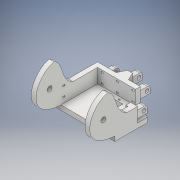
# Autodesk Inventor part: palm
Saved by Autodesk Inventor 2018 (Build 220112000, 112)
## iProperties
Created: 2018-02-09
Part Number: palm
Material: Plastique ABS
Document SubType Name: Modeling
Designer: Thomas
Density: 1.06 g/cm^3
Appearance: Lisse - Blanc
Author: Thomas
Autodesk Inventor part; units mm, degrees
ref_plane "YZ Plane" through (0, 0, 0) normal (1, 0, 0) x (0, 1, 0)
ref_plane "XZ Plane" through (0, 0, 0) normal (0, 1, 0) x (-1, 0, 0)
ref_plane "XY Plane" through (0, 0, 0) normal (0, 0, 1) x (1, 0, 0)
sketch "Esquisse1" plane through (0, 0, 0) normal (0, 0, 1) x (1, 0, 0)
  line L0 (0, 0) -> (44.9, 0)
  line L1 (44.9, 0) -> (44.9, 5)
  line L2 (0, 5) -> (0, 0)
  line L3 (23.4, 13) -> (28.6, 13)
  line L4 (28.6, 13) -> (32.5, 5)
  line L5 (23.4, 13) -> (19.5, 5)
  line L6 (0, 5) -> (19.5, 5)
  line L7 (32.5, 5) -> (44.9, 5)
  line L8 (28.6, 13) -> (28.6, 5) construction
  line L9 (28.6, 5) -> (32.5, 5) construction
  line L10 (23.4, 13) -> (23.4, 5) construction
  line L11 (23.4, 5) -> (19.5, 5) construction
  dimension "d0" = 5
  dimension "d1" = 44.9
  dimension "d2" = 13
  dimension "d3" = 13
  dimension "d5" = 5.2
  dimension "d146" = 3.9
  dimension "d147" = 3.9
  dimension "d148" = 12.4
  constraints: 24 end point, 4 horizontal, 2 perpendicular, 1 collinear, 1 parallel, 1 vertical
  measures "d0" distance of L0.end L1.end
  measures "d1" distance of L1.end L2.start
  measures "d2" distance of L4.end L5.end
  measures "d3" distance between parallel lines of L0 L3
  measures "d5" distance of L3.start L3.end
  measures "d146" distance of L8.end L4.end
  measures "d147" distance of L10.end L5.end
  measures "d148" distance of L4.end L1.end
extrude "Extrusion1" add sketch "Esquisse1" along normal blind 15
sketch "Esquisse2" plane through (44.9, 0, 0) normal (1, 0, 0) x (0, 0, -1)
  line L0 (0, 0) -> (-15, 0) projected
  line L1 (0, 0) -> (-15, 0)
  line L2 (-15, 0) -> (-15, -19.5)
  line L3 (-15, -19.5) -> (0, -19.5)
  line L4 (0, -19.5) -> (0, 0)
  point P0 (-15, 5)
  dimension "d11" = 19.5
  dimension "d18" = 15
  constraints: 8 end point, 2 parallel, 1 horizontal, 1 perpendicular
  measures "d11" distance of L3.end L0.start
  measures "d18" distance of L2.end L3.end
extrude "Extrusion2" add sketch "Esquisse2" against normal blind 5
sketch "Esquisse3" plane through (44.9, -19.5, 0) normal (0, -1, 0) x (1, 0, 0)
  line L0 (0, 0) -> (0, 15) projected
  line L1 (0, 15) -> (16.5, 15)
  line L2 (16.5, 15) -> (16.5, 0)
  line L3 (16.5, 0) -> (0, 0)
  line L4 (0, 0) -> (0, 15)
  point P0 (-44.9, 0)
  dimension "d14" = 16.5
  dimension "d19" = 15
  constraints: 8 end point, 2 parallel, 1 horizontal, 1 perpendicular
  measures "d14" distance of L2.end L3.end
  measures "d19" distance of L1.end L2.end
extrude "Extrusion3" add sketch "Esquisse3" against normal blind 5
sketch "Esquisse5" plane through (61.4, -19.5, 15) normal (1, 0, 0) x (0, 0, -1)
  line L0 (0, 0) -> (0, 19.5) projected
  spline S0 degree 3 poles (15, -18.85) (12.4289, -60.7765) (-25.3218, -44.0983) (-27.81, -26.0736) knots 0 0 0 0 1 1 1 1
  line L1 (0, 0) -> (-12.0102, 0) construction
  spline S1 degree 3 poles (0, -6.5) (-6.4739, -20.1212) (-23.0066, -15.548) (-27.81, -26.0736) knots 0 0 0 0 1 1 1 1
  line L2 (15, 0) -> (0, 0)
  line L3 (15, 19.5) -> (15, 0) projected
  line L4 (15, -18.85) -> (15, 0)
  line L5 (15, 0) -> (0, 0) projected
  line L6 (15, 0) -> (0, 0)
  line L7 (0, 0) -> (0, -6.5)
  line L8 (0, -26) -> (-10, -26) construction
  circle A0 centre (-5, -26) radius 5 construction
  point P0 (-0.0048, -44.59)
  point P1 (-18.0068, -40.3478)
  point P2 (-9.9873, -15.735)
  point P3 (-20.8554, -19.7545)
  dimension "d21" = 6.5
  dimension "d24" = 10
  dimension "d26" = 26
  dimension "d27" = 26
  dimension "d28" = 44.59
  dimension "d31" = 17.81
  dimension "d32" = 10
  constraints: 12 end point, 2 horizontal, 1 centre point, 1 collinear, 1 midpoint, 1 perpendicular, 1 vertical, 8 other
  measures "d21" distance of L0.start L7.end
  measures "d24" distance of L8.end L8.start
  measures "d26" distance of L0.start L8.start
  measures "d27" distance from line of L1 L8.end
  measures "d28" distance of point (-0.005, -44.59) L0.start
  measures "d31" horizontal distance of point (-27.81, -26.074) L8.end
  measures "d32" diameter of A0
extrude "Extrusion4" add sketch "Esquisse5" against normal blind 5
sketch "Esquisse6" plane through (61.4, -14.5, 15) normal (1, 0, 0) x (0, 0, -1)
  circle A0 centre (-5.6857, -35.9029) radius 2.6
  point P0 (15, 14.5)
  point P1 (0, 0)
  dimension "d213" = 5.2
  constraints: 1 centre point, 1 coincident
  measures "d213" diameter of A0
extrude "Extrusion5" cut sketch "Esquisse6" against normal blind 5
sketch "Esquisse7" plane through (0, 0, 0) normal (-1, 0, 0) x (0, 0, 1)
  line L0 (15, -19.4715) -> (15, 0)
  spline S0 degree 3 poles (0, -38.3215) (2.8582, -79.9664) (39.8923, -64.0148) (42.81, -45.5451) knots 0 0 0 0 1 1 1 1
  line L1 (15, -19.4715) -> (27.0102, -19.4715) construction
  spline S1 degree 3 poles (15, -25.9715) (21.48, -39.5796) (38.0003, -35.0338) (42.81, -45.5451) knots 0 0 0 0 1 1 1 1
  line L2 (0, 0) -> (0, -19.4715)
  line L3 (0, -38.3215) -> (0, -19.4715)
  line L4 (15, -19.4715) -> (15, -25.9715)
  line L5 (15, -45.4715) -> (25, -45.4715) construction
  circle A0 centre (20, -45.4715) radius 5 construction
  line L6 (15, 0) -> (0, 0)
  line L7 (0, 0) -> (15, 0) projected
  line L8 (15, -19.5) -> (15, 0) projected
  line L9 (0, 0) -> (0, -19.5) projected
  line L10 (0, -19.5) -> (15, -19.5) construction
  line L11 (15, -19.5) -> (15, -70.8185) construction
  point P0 (15, -26)
  point P1 (15, -64.0615)
  point P2 (32.7077, -60.0762)
  point P3 (24.9887, -35.2044)
  point P4 (35.8544, -39.2301)
  point P5 (42.81, -45.5736)
  dimension "d62" = 0
  dimension "d63" = 0
  dimension "d64" = 0
  dimension "d66" = 17.81
  dimension "d67" = 44.59
  dimension "d68" = 0
  dimension "d69" = 10
  dimension "d70" = 5
  dimension "d71" = 0
  constraints: 16 end point, 1 centre point, 1 horizontal, 1 vertical, 8 other
  measures "d62" distance between parallel lines of L7 L6
  measures "d63" distance between parallel lines of L0 L8
  measures "d64" distance between parallel lines of L2 L9
  measures "d66" horizontal distance of point (42.81, -45.545) L5.end
  measures "d67" distance of point (15, -64.062) L1.start
  measures "d68" distance from line of L11 L5.start
  measures "d69" diameter of A0
  measures "d70" distance of L5.start A0.centre
  measures "d71" distance from line of L11 point (15, -64.062)
extrude "Extrusion6" add sketch "Esquisse7" against normal blind 5
sketch "Esquisse9" plane through (0, 5, 0) normal (-1, 0, 0) x (0, 0, 1)
  line L0 (0, 0) -> (15, 0) construction
  line L1 (15, 0) -> (15, -38) construction
  line L2 (15, -38) -> (7.2, -38)
  line L3 (7.2, -38) -> (7.2, -43.2)
  line L4 (7.2, -43.2) -> (15, -43.2)
  line L5 (15, -43.2) -> (15, -38)
  point P0 (0, -5)
  dimension "d76" = 38
  dimension "d78" = 7.8
  dimension "d79" = 5.2
  constraints: 10 end point, 2 vertical, 1 horizontal, 1 parallel, 1 perpendicular
  measures "d76" distance of L0.end L1.end
  measures "d78" distance of L1.end L2.end
  measures "d79" distance of L2.end L3.end
extrude "Extrusion8" add sketch "Esquisse9" along normal blind 10.4
sketch "Esquisse10" plane through (0, -33, 15) normal (0, 1, 0) x (1, 0, 0)
  circle A0 centre (-6.9337, 3.9) radius 2
  arc A1 (-10.4, 3) -> (-7.4, 0) centre (-7.4, 3) ccw construction
  line L0 (-10.4, 3) -> (-10.4, 10.1049) construction
  line L1 (-10.4, 10.1049) -> (-10.4, -0.5302) construction
  line L2 (0, 0) -> (-10.4, 0) construction
  line L3 (0, 7.8) -> (0, 0) construction
  line L4 (0, 7.8) -> (-10.4, 7.8) construction
  line L5 (-3.4673, 0) -> (-3.4673, 7.8) construction
  line L6 (-10.4, 0) -> (-3.4673, 7.8) construction
  line L7 (-3.4673, 0) -> (-10.4, 7.8) construction
  point P0 (0, 15)
  dimension "d84" = 4
  dimension "d111" = 3.4674
  constraints: 14 end point, 5 point on line, 3 perpendicular, 1 centre point, 1 midpoint, 1 point on circle, 1 tangent, 1 vertical
  measures "d84" diameter of A0
  measures "d111" distance between parallel lines of L3 L5
extrude "Extrusion9" cut sketch "Esquisse10" against normal blind 5.2
sketch "Esquisse11" plane through (0, 5, 0) normal (-1, 0, 0) x (0, 0, 1)
  line L0 (11.1472, -39.2716) -> (11.1472, -43.1725)
  line L1 (7.2, -38) -> (15, -38) projected
  line L2 (14.1279, -41.7) -> (14.1279, -39.5)
  line L3 (15, -38) -> (15, -43.2) projected
  line L4 (17, -41.7) -> (15.5, -41.7)
  line L5 (15.5, -41.7) -> (15.5, -39.5)
  line L6 (15.5, -39.5) -> (17, -39.5)
  line L7 (17, -39.5) -> (17, -41.7)
  line L8 (6.7, -41.7) -> (5.2, -41.7)
  line L9 (5.2, -41.7) -> (5.2, -39.5)
  line L10 (5.2, -39.5) -> (6.7, -39.5)
  line L11 (6.7, -39.5) -> (6.7, -41.7)
  line L12 (7.2, -43.2) -> (7.2, -38) projected
  point P0 (0, -5)
  dimension "d93" = 0.5
  dimension "d94" = 1.5
  dimension "d95" = 1.5
  dimension "d96" = 2.2
  dimension "d97" = 2.2
  dimension "d98" = 1.5
  dimension "d99" = 0.5
  dimension "d100" = 1.5
  constraints: 20 end point, 4 parallel, 2 horizontal, 2 perpendicular
  measures "d93" distance between parallel lines of L3 L5
  measures "d94" distance of L5.end L6.end
  measures "d95" distance between parallel lines of L6 L1
  measures "d96" distance of L6.end L4.start
  measures "d97" distance of L8.end L9.end
  measures "d98" distance of L9.end L10.end
  measures "d99" distance between parallel lines of L12 L11
  measures "d100" distance between parallel lines of L1 L10
extrude "Extrusion11" cut sketch "Esquisse11" against normal blind 5
sketch "Esquisse12" plane through (0, 5, 0) normal (0, 1, 0) x (1, 0, 0)
  line L0 (7.15, -11.4) -> (12.35, -11.4)
  line L1 (12.35, -11.4) -> (12.35, -3.6)
  line L2 (12.35, -3.6) -> (7.15, -3.6)
  line L3 (7.15, -3.6) -> (7.15, -11.4)
  line L4 (19.5, 0) -> (0, 0) projected
  line L5 (0, 0) -> (0, -15) projected
  dimension "d103" = 7.8
  dimension "d104" = 5.2
  dimension "d105" = 3.6
  dimension "d106" = 7.15
  constraints: 8 end point, 2 parallel, 1 horizontal, 1 perpendicular
  measures "d103" distance of L2.end L0.start
  measures "d104" distance of L0.start L0.end
  measures "d105" distance between parallel lines of L4 L2
  measures "d106" distance between parallel lines of L5 L3
extrude "Extrusion12" add sketch "Esquisse12" along normal blind 10.4
fillet "Congé2" radius 3 1 edges at (9.75, 15.4, 11.4)
fillet "Congé3" radius 3 1 edges at (-10.4, -35.6, 15)
sketch "Esquisse13" plane through (7.15, 5, 3.6) normal (-1, 0, 0) x (0, 0, 1)
  line L0 (7.8, 0) -> (7.8, 7.4) construction
  line L1 (7.8, 0) -> (7.8, 11.1767) construction
  line L2 (7.8, 0) -> (0, 0) construction
  line L3 (0, 0) -> (0, 11.2768) construction
  line L4 (0, 0) -> (0, 10.4) construction
  line L5 (0, 10.4) -> (7.8, 10.4) construction
  line L6 (7.8, 3.467) -> (0, 3.467) construction
  line L7 (0, 3.467) -> (7.8, 10.4) construction
  line L8 (7.8, 3.467) -> (0, 10.4) construction
  circle A0 centre (3.9, 6.9335) radius 2
  point P0 (-3.6, -5)
  dimension "d113" = 3.467
  dimension "d114" = 4
  constraints: 12 end point, 4 point on line, 1 centre point, 1 horizontal, 1 midpoint, 1 perpendicular, 1 vertical
  measures "d113" distance between parallel lines of L2 L6
  measures "d114" diameter of A0
extrude "Extrusion13" cut sketch "Esquisse13" against normal blind 5.2
sketch "Esquisse16" plane through (0, 5, 0) normal (0, 1, 0) x (1, 0, 0)
  line L0 (10.85, -13.4) -> (8.65, -13.4)
  line L1 (8.65, -13.4) -> (8.65, -11.9)
  line L2 (8.65, -11.9) -> (10.85, -11.9)
  line L3 (10.85, -11.9) -> (10.85, -13.4)
  line L4 (10.85, -3.1) -> (8.65, -3.1)
  line L5 (8.65, -3.1) -> (8.65, -1.6)
  line L6 (8.65, -1.6) -> (10.85, -1.6)
  line L7 (10.85, -1.6) -> (10.85, -3.1)
  line L8 (12.35, -11.4) -> (7.15, -11.4) projected
  line L9 (7.15, -11.4) -> (7.15, -3.6) projected
  line L10 (7.15, -3.6) -> (12.35, -3.6) projected
  point P0 (0, 0)
  dimension "d117" = 2.2
  dimension "d118" = 2.2
  dimension "d119" = 1.5
  dimension "d120" = 1.5
  dimension "d121" = 0.5
  dimension "d122" = 1.5
  dimension "d123" = 0.5
  constraints: 16 end point, 4 parallel, 2 horizontal, 2 perpendicular, 1 point on line
  measures "d117" distance of L5.end L6.end
  measures "d118" distance of L1.end L2.end
  measures "d119" distance of L4.end L5.end
  measures "d120" distance of L0.end L1.end
  measures "d121" distance between parallel lines of L8 L2
  measures "d122" distance between parallel lines of L9 L1
  measures "d123" distance between parallel lines of L10 L4
extrude "Extrusion14" cut sketch "Esquisse16" against normal blind 5
sketch "Esquisse18" plane through (23.4, 13, 0) normal (0, 1, 0) x (1, 0, 0)
  line L0 (5.2, 0) -> (5.2, -15) construction
  line L1 (5.2, 0) -> (0, 0) construction
  line L2 (5.2, 0) -> (0, 0) construction
  line L3 (5.2, -15) -> (0, -15) construction
  line L4 (0, 0) -> (0, -15) construction
  line L5 (0, -15) -> (5.2, -15) construction
  line L6 (0, 0) -> (0, -15) projected
  line L7 (5.2, -11.4) -> (0, -11.4)
  line L8 (0, -11.4) -> (0, -3.6)
  line L9 (0, -3.6) -> (5.2, -3.6)
  line L10 (5.2, -3.6) -> (5.2, -11.4)
  point P0 (-23.4, 0)
  dimension "d126" = 7.8
  dimension "d128" = 3.6
  constraints: 14 end point, 4 equal length, 2 perpendicular, 2 point on line, 1 horizontal
  measures "d126" distance of L7.end L8.end
  measures "d128" distance between parallel lines of L1 L9
extrude "Extrusion15" add sketch "Esquisse18" along normal blind 10.4
fillet "Congé4" radius 3 1 edges at (26, 23.4, 11.4)
sketch "Esquisse19" plane through (23.4, 13, 15) normal (0, 1, 0) x (1, 0, 0)
  line L0 (3.7, 1.6) -> (1.5, 1.6)
  line L1 (1.5, 1.6) -> (1.5, 3.1)
  line L2 (1.5, 3.1) -> (3.7, 3.1)
  line L3 (3.7, 3.1) -> (3.7, 1.6)
  line L4 (3.7, 11.9) -> (1.5, 11.9)
  line L5 (1.5, 11.9) -> (1.5, 13.4)
  line L6 (1.5, 13.4) -> (3.7, 13.4)
  line L7 (3.7, 13.4) -> (3.7, 11.9)
  line L8 (5.2, 3.6) -> (0, 3.6) projected
  line L9 (0, 11.4) -> (5.2, 11.4) projected
  line L10 (0, 11.4) -> (0, 3.6) projected
  point P0 (-23.4, 15)
  dimension "d132" = 1.5
  dimension "d133" = 2.2
  dimension "d134" = 1.5
  dimension "d135" = 0.5
  dimension "d136" = 0.5
  dimension "d137" = 1.5
  constraints: 16 end point, 4 parallel, 2 horizontal, 2 perpendicular, 2 point on line
  measures "d132" distance of L2.end L0.start
  measures "d133" distance of L1.end L2.end
  measures "d134" distance of L6.end L4.start
  measures "d135" distance between parallel lines of L8 L2
  measures "d136" distance between parallel lines of L9 L4
  measures "d137" distance between parallel lines of L10 L5
extrude "Extrusion16" cut sketch "Esquisse19" against normal blind 20
sketch "Esquisse20" plane through (28.6, 13, 3.6) normal (1, 0, 0) x (0, 0, -1)
  line L0 (0, 0) -> (0, 10.4) construction
  line L1 (0, 0) -> (0, 10.4) construction
  line L2 (0, 10.4) -> (-8.133, 10.213) construction
  line L3 (0, 0) -> (-7.8, 0) construction
  line L4 (-7.8, 0) -> (0, 0) construction
  line L5 (-7.8, 0) -> (-7.8, 10.2207) construction
  line L6 (-7.8, 3.467) -> (0, 3.467) construction
  line L7 (-7.8, 3.467) -> (0, 10.4) construction
  line L8 (0, 3.467) -> (-7.8, 10.2207) construction
  circle A0 centre (-3.9, 6.8438) radius 2
  point P0 (3.6, -13)
  dimension "d140" = 3.467
  dimension "d141" = 4
  constraints: 14 end point, 3 point on line, 2 vertical, 1 centre point, 1 horizontal, 1 midpoint, 1 perpendicular
  measures "d140" distance between parallel lines of L4 L6
  measures "d141" diameter of A0
extrude "Extrusion17" cut sketch "Esquisse20" against normal blind 5.2
sketch "Esquisse21" plane through (32.5, 5, 0) normal (0, 1, 0) x (1, 0, 0)
  line L0 (12.35, -11.4) -> (7.15, -11.4)
  line L1 (7.15, -11.4) -> (7.15, -3.6)
  line L2 (7.15, -3.6) -> (12.35, -3.6)
  line L3 (12.35, -3.6) -> (12.35, -11.4)
  line L4 (0, 0) -> (0, -15) projected
  line L5 (12.4, 0) -> (0, 0) projected
  point P0 (-32.5, 0)
  dimension "d144" = 5.2
  dimension "d145" = 7.8
  dimension "d149" = 7.15
  dimension "d150" = 3.6
  constraints: 8 end point, 2 parallel, 1 horizontal, 1 perpendicular
  measures "d144" distance of L0.start L0.end
  measures "d145" distance of L0.end L1.end
  measures "d149" distance between parallel lines of L4 L1
  measures "d150" distance between parallel lines of L5 L2
extrude "Extrusion18" add sketch "Esquisse21" along normal blind 10.4
fillet "Congé5" radius 3 1 edges at (42.25, 15.4, 11.4)
sketch "Esquisse22" plane through (44.85, 5, 11.4) normal (1, 0, 0) x (0, 0, -1)
  line L0 (0, 0) -> (7.8, 0) construction
  line L1 (7.8, 0) -> (7.8, 10.4) construction
  line L2 (7.8, 0) -> (7.8, 10.4) construction
  line L3 (7.8, 10.4) -> (0, 10.4) construction
  line L4 (0, 0) -> (0, 7.4) construction
  line L5 (0, 10.4) -> (0, 0) construction
  line L6 (0, 3.467) -> (7.8, 3.467) construction
  line L7 (3, 10.4) -> (7.8, 10.4) construction
  line L8 (0, 3.467) -> (7.8, 10.4) construction
  line L9 (0, 10.4) -> (7.8, 3.467) construction
  circle A0 centre (3.9, 6.9335) radius 2
  point P0 (11.4, -5)
  dimension "d154" = 3.467
  dimension "d155" = 4
  constraints: 12 end point, 2 collinear, 2 perpendicular, 2 point on line, 1 centre point, 1 midpoint
  measures "d154" distance between parallel lines of L6 L0
  measures "d155" diameter of A0
extrude "Extrusion19" cut sketch "Esquisse22" against normal blind 5.2
sketch "Esquisse23" plane through (32.5, 5, 0) normal (0, 1, 0) x (1, 0, 0)
  line L0 (10.85, -13.4) -> (8.65, -13.4)
  line L1 (8.65, -13.4) -> (8.65, -11.9)
  line L2 (8.65, -11.9) -> (10.85, -11.9)
  line L3 (10.85, -11.9) -> (10.85, -13.4)
  line L4 (10.85, -3.1) -> (8.65, -3.1)
  line L5 (8.65, -3.1) -> (8.65, -1.6)
  line L6 (8.65, -1.6) -> (10.85, -1.6)
  line L7 (10.85, -1.6) -> (10.85, -3.1)
  line L8 (12.35, -11.4) -> (7.15, -11.4) projected
  line L9 (7.15, -11.4) -> (7.15, -3.6) projected
  line L10 (7.15, -3.6) -> (12.35, -3.6) projected
  point P0 (-32.5, 0)
  dimension "d158" = 2.2
  dimension "d159" = 1.5
  dimension "d160" = 0.5
  dimension "d161" = 1.5
  dimension "d162" = 1.5
  dimension "d163" = 0.5
  constraints: 16 end point, 4 parallel, 2 horizontal, 2 perpendicular, 2 point on line
  measures "d158" distance of L1.end L2.end
  measures "d159" distance of L0.end L1.end
  measures "d160" distance between parallel lines of L2 L8
  measures "d161" distance between parallel lines of L9 L1
  measures "d162" distance of L4.end L5.end
  measures "d163" distance between parallel lines of L10 L4
extrude "Extrusion20" cut sketch "Esquisse23" against normal blind 24.5
sketch "Esquisse24" plane through (44.9, -14.5, 0) normal (0, 1, 0) x (1, 0, 0)
  line L0 (16.25, -11.4) -> (11.05, -11.4)
  line L1 (11.05, -11.4) -> (11.05, -3.6)
  line L2 (11.05, -3.6) -> (16.25, -3.6)
  line L3 (16.25, -3.6) -> (16.25, -11.4)
  line L4 (0, 0) -> (0, -15) projected
  line L5 (16.5, 0) -> (0, 0) projected
  point P0 (-44.9, 0)
  dimension "d166" = 7.8
  dimension "d167" = 5.2
  dimension "d168" = 11.05
  dimension "d169" = 3.6
  constraints: 8 end point, 2 parallel, 1 horizontal, 1 perpendicular
  measures "d166" distance of L0.end L1.end
  measures "d167" distance of L0.start L0.end
  measures "d168" distance between parallel lines of L4 L1
  measures "d169" distance between parallel lines of L5 L2
extrude "Extrusion21" add sketch "Esquisse24" along normal blind 10.4
fillet "Congé6" radius 3 1 edges at (58.55, -4.1, 11.4)
sketch "Esquisse25" plane through (61.15, -14.5, 11.4) normal (1, 0, 0) x (0, 0, -1)
  line L0 (7.8, 0) -> (7.8, 10.4) construction
  line L1 (0, 0) -> (7.8, 0) construction
  line L2 (7.8, 0) -> (7.8, 10.4) construction
  line L3 (7.8, 10.4) -> (0, 10.4) construction
  line L4 (0, 0) -> (0, 7.4) construction
  line L5 (0, 10.4) -> (0, 0) construction
  line L6 (0, 3.467) -> (7.8, 3.467) construction
  line L7 (7.8, 0) -> (7.8, 10.4) construction
  line L8 (0, 0) -> (7.8, 0) construction
  line L9 (0, 3.467) -> (7.8, 10.4) construction
  line L10 (0, 10.4) -> (7.8, 3.467) construction
  circle A0 centre (3.9, 6.9335) radius 2
  point P0 (11.4, 14.5)
  dimension "d173" = 3.467
  dimension "d174" = 4
  constraints: 14 end point, 2 collinear, 2 horizontal, 2 point on line, 1 centre point, 1 midpoint, 1 perpendicular
  measures "d173" distance between parallel lines of L8 L6
  measures "d174" diameter of A0
extrude "Extrusion22" cut sketch "Esquisse25" against normal blind 5.2
sketch "Esquisse26" plane through (44.9, -14.5, 0) normal (0, 1, 0) x (1, 0, 0)
  line L0 (14.75, -3.1) -> (12.55, -3.1)
  line L1 (12.55, -3.1) -> (12.55, -1.6)
  line L2 (12.55, -1.6) -> (14.75, -1.6)
  line L3 (14.75, -1.6) -> (14.75, -3.1)
  line L4 (14.75, -13.4) -> (12.55, -13.4)
  line L5 (12.55, -13.4) -> (12.55, -11.9)
  line L6 (12.55, -11.9) -> (14.75, -11.9)
  line L7 (14.75, -11.9) -> (14.75, -13.4)
  line L8 (16.25, -11.4) -> (11.05, -11.4) projected
  line L9 (11.05, -11.4) -> (11.05, -3.6) projected
  line L10 (11.05, -3.6) -> (16.25, -3.6) projected
  point P0 (-44.9, 0)
  dimension "d177" = 2.2
  dimension "d178" = 2.2
  dimension "d179" = 0.5
  dimension "d180" = 1.5
  dimension "d181" = 1.5
  dimension "d182" = 0.5
  dimension "d183" = 1.5
  constraints: 16 end point, 4 parallel, 2 horizontal, 2 perpendicular, 1 point on line
  measures "d177" distance of L1.end L2.end
  measures "d178" distance of L4.start L4.end
  measures "d179" distance between parallel lines of L6 L8
  measures "d180" distance of L4.end L5.end
  measures "d181" distance between parallel lines of L9 L5
  measures "d182" distance between parallel lines of L10 L0
  measures "d183" distance of L0.end L1.end
extrude "Extrusion23" cut sketch "Esquisse26" against normal blind 10
sketch "Esquisse27" plane through (56.4, -19.5, 15) normal (-1, 0, 0) x (0, 0, 1)
  line L0 (-1.6, -5) -> (-3.1, -5)
  line L1 (-3.1, -5) -> (-3.1, -2.8)
  line L2 (-3.1, -2.8) -> (-1.6, -2.8)
  line L3 (-1.6, -2.8) -> (-1.6, -5)
  line L4 (-11.9, -5) -> (-13.4, -5)
  line L5 (-13.4, -5) -> (-13.4, -2.8)
  line L6 (-13.4, -2.8) -> (-11.9, -2.8)
  line L7 (-11.9, -2.8) -> (-11.9, -5)
  line L8 (-15, 0) -> (0, 0) projected
  line L9 (-15, 0) -> (-15, -18.85) projected
  point P0 (-15, 19.5)
  dimension "d186" = 2.2
  dimension "d187" = 1.5
  dimension "d188" = 2.8
  dimension "d189" = 8.8
  dimension "d190" = 1.5
  dimension "d191" = 1.6
  constraints: 16 end point, 4 parallel, 2 horizontal, 2 perpendicular, 2 point on line
  measures "d186" distance of L2.end L0.start
  measures "d187" distance of L1.end L2.end
  measures "d188" distance between parallel lines of L8 L2
  measures "d189" distance between parallel lines of L7 L1
  measures "d190" distance of L5.end L6.end
  measures "d191" distance between parallel lines of L9 L5
extrude "Extrusion24" cut sketch "Esquisse27" against normal blind 3
sketch "Esquisse29" plane through (0, 0, 0) normal (0, 0, -1) x (-1, 0, 0)
  line L0 (0, -38.3215) -> (-5, -38.3215) projected
  line L1 (-61.4, -38.35) -> (-56.4, -38.35) projected
  line L2 (0, -38.3215) -> (-61.4, -38.35)
  line L3 (-61.4, -38.35) -> (-61.4, -4.1)
  line L4 (-61.4, -4.1) -> (-40.2696, 5)
  line L5 (-19.5, 5) -> (0, 5) projected
  line L6 (0, 5) -> (-40.2696, 5)
  line L7 (0, 5) -> (0, -38.3215) projected
  line L8 (0, -38.3215) -> (0, 5)
  point P0 (0, 0)
  constraints: 10 end point, 2 vertical, 1 collinear
extrude "Extrusion25" add sketch "Esquisse29" along normal blind 5
sketch "Esquisse30" plane through (0, 0, 15) normal (0, 0, 1) x (1, 0, 0)
  line L0 (39.9, -19.5) -> (56.4, -19.5) projected
  line L1 (54.1535, -19.5) -> (54.1535, 0)
  line L2 (5, 0) -> (39.9, 0) projected
  line L3 (54.1535, 0) -> (39.9, 0)
  line L4 (39.9, -19.5) -> (39.9, 0) projected
  line L5 (39.9, 0) -> (39.9, -19.5)
  line L6 (39.9, -19.5) -> (54.1535, -19.5)
  point P0 (0, 0)
  constraints: 8 end point, 2 perpendicular, 1 collinear, 1 point on line, 1 vertical
extrude "Extrusion26" cut sketch "Esquisse30" against normal blind 15
sketch "Esquisse31" plane through (0, 0, -5) normal (0, 0, -1) x (-1, 0, 0)
  line L0 (-61.4, -4.1) -> (-61.4, -38.35) construction
  line L1 (0, -38.2) -> (10.4, -38.2) construction
  line L2 (-61.4, -38.35) -> (0, -38.2) construction
  line L3 (0, 5) -> (0, -25.9715) construction
  line L4 (0, -38.2) -> (0, 5) construction
  line L5 (0, 5) -> (-61.4, 5) construction
  line L6 (-61.4, 5) -> (-61.4, -38.35) construction
  line L7 (-36.7, -5) -> (-24.7, -5)
  line L8 (-24.7, -5) -> (-24.7, -28)
  line L9 (-24.7, -28) -> (-36.7, -28)
  line L10 (-36.7, -28) -> (-36.7, -5)
  line L11 (-31.7, -2.5) -> (-29.7, -2.5)
  line L12 (-29.7, -2.5) -> (-29.7, -3.5)
  line L13 (-29.7, -3.5) -> (-31.7, -3.5)
  line L14 (-31.7, -3.5) -> (-31.7, -2.5)
  line L15 (-31.7, -29.5) -> (-29.7, -29.5)
  line L16 (-29.7, -29.5) -> (-29.7, -30.5)
  line L17 (-29.7, -30.5) -> (-31.7, -30.5)
  line L18 (-31.7, -30.5) -> (-31.7, -29.5)
  point P0 (0, 0)
  dimension "d199" = 12
  dimension "d200" = 23
  dimension "d203" = 2
  dimension "d204" = 1
  dimension "d205" = 1.5
  dimension "d206" = 2
  dimension "d207" = 1
  dimension "d208" = 1.5
  dimension "d209" = 5
  dimension "d212" = 10
  constraints: 32 end point, 6 parallel, 5 perpendicular, 3 horizontal, 1 collinear, 1 point on line
  measures "d199" distance of L8.end L9.end
  measures "d200" distance of L7.end L8.end
  measures "d203" distance of L16.end L17.end
  measures "d204" distance of L15.end L16.end
  measures "d205" distance between parallel lines of L9 L15
  measures "d206" distance of L11.start L11.end
  measures "d207" distance of L11.end L12.end
  measures "d208" distance between parallel lines of L7 L13
  measures "d209" distance between parallel lines of L8 L12
  measures "d212" distance between parallel lines of L7 L5
extrude "Extrusion27" cut sketch "Esquisse31" against normal blind 5
sketch "Esquisse32" plane through (0, -25.9715, 15) normal (-1, 0, 0) x (0, 0, 1)
  circle A0 centre (5.6857, -24.4314) radius 2.6 projected
  circle A1 centre (5.6857, -24.4314) radius 2.6
  point P0 (-15, 25.9715)
  constraints: 2 coincident, 1 centre point, 1 concentric
extrude "Extrusion28" cut sketch "Esquisse32" against normal blind 5
